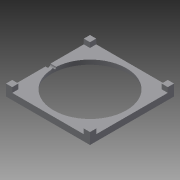
# Autodesk Inventor part: lamp_holder_v1
Saved by Autodesk Inventor 2015 (Build 190159000, 159)
## iProperties
Created: 2021-08-24
Part Number: lamp_holder_v1
Material: Genérico
Document SubType Name: Modeling
Designer: Zuloaga
Density: 1 g/cm^3
Appearance: Valor por defecto
Author: Zuloaga
Autodesk Inventor part; units mm, degrees
ref_plane "YZ Plane" through (0, 0, 0) normal (1, 0, 0) x (0, 1, 0)
ref_plane "XZ Plane" through (0, 0, 0) normal (0, 1, 0) x (-1, 0, 0)
ref_plane "XY Plane" through (0, 0, 0) normal (0, 0, 1) x (1, 0, 0)
sketch "Boceto1" plane through (0, 0, 0) normal (0, 0, 1) x (1, 0, 0)
  circle A0 centre (0, 0) radius 62.5
  line L0 (62.5, 0) -> (67.5, 0)
  line L1 (0, 62.5) -> (0, 67.5)
  line L2 (0, 62.5) -> (5, 62.5) construction
  line L3 (0, 67.5) -> (67.5, 67.5)
  line L4 (67.5, 67.5) -> (67.5, 0)
  line L5 (-62.5, 0) -> (-67.5, 0)
  line L6 (-62.5, 0) -> (-57.5, 0) construction
  line L7 (0, -62.5) -> (0, -67.5)
  line L8 (0, -62.5) -> (5, -62.5) construction
  line L9 (0, -67.5) -> (-67.5, -67.5)
  line L10 (-67.5, -67.5) -> (67.5, -67.5)
  line L11 (67.5, -67.5) -> (67.5, 67.5)
  line L12 (67.5, 67.5) -> (-67.5, 67.5)
  line L13 (-67.5, 67.5) -> (-67.5, -67.5)
  dimension "d0" = 125
  dimension "d1" = 5
  dimension "d2" = 5
  dimension "d3" = 90
  dimension "d4" = 90
  dimension "d5" = 5
  dimension "d6" = 180
  dimension "d7" = 5
  dimension "d8" = 90
  dimension "d9" = 90
  constraints: 28 end point, 6 horizontal, 4 point on circle, 3 equal length, 2 parallel, 2 perpendicular, 2 vertical, 1 centre point, 1 coincident
  measures "d0" diameter of A0
  measures "d1" distance of L0.start L0.end
  measures "d2" distance of L1.start L1.end
  measures "d3" angle of L2 L1
  measures "d4" angle of L1 L3
  measures "d5" distance of L5.start L5.end
  measures "d6" angle of L5 L6
  measures "d7" distance of L7.start L7.end
  measures "d8" angle of L7 L8
  measures "d9" angle of L7 L9
extrude "Extrusión1" add sketch "Boceto1" along normal blind 7 contours L0 L11 L10 L7 A0 | A0 L1 L3 L4 L0 | A0 L5 L13 L12 L1 | L7 L9 L13 L5 A0
sketch "Boceto2" plane through (0, 0, 7) normal (0, 0, 1) x (1, 0, 0)
  line L0 (-67.5, 67.5) -> (67.5, 67.5)
  line L1 (67.5, 67.5) -> (67.5, -67.5)
  line L2 (67.5, -67.5) -> (-67.5, -67.5)
  line L3 (-67.5, -67.5) -> (-67.5, 67.5)
  circle A0 centre (0, 0) radius 58.5
  dimension "d12" = 117
  constraints: 8 end point, 2 parallel, 1 centre point, 1 coincident, 1 horizontal, 1 perpendicular
  measures "d12" diameter of A0
extrude "Extrusión2" add sketch "Boceto2" along normal blind 3
sketch "Boceto3" plane through (0, 0, 10) normal (0, 0, 1) x (1, 0, 0)
  line L0 (-67.5, -67.5) -> (-57.5, -67.5)
  line L1 (-57.5, -67.5) -> (-57.5, -57.5)
  line L2 (-57.5, -57.5) -> (-67.5, -57.5)
  line L3 (-67.5, -57.5) -> (-67.5, -67.5)
  line L4 (67.5, 67.5) -> (57.5, 67.5)
  line L5 (57.5, 67.5) -> (57.5, 57.5)
  line L6 (57.5, 57.5) -> (67.5, 57.5)
  line L7 (67.5, 57.5) -> (67.5, 67.5)
  line L8 (-67.5, 67.5) -> (-57.5, 67.5)
  line L9 (-57.5, 67.5) -> (-57.5, 57.5)
  line L10 (-57.5, 57.5) -> (-67.5, 57.5)
  line L11 (-67.5, 57.5) -> (-67.5, 67.5)
  line L12 (67.5, -67.5) -> (57.5, -67.5)
  line L13 (57.5, -67.5) -> (57.5, -57.5)
  line L14 (57.5, -57.5) -> (67.5, -57.5)
  line L15 (67.5, -57.5) -> (67.5, -67.5)
  point P0 (0, 0)
  dimension "d15" = 10
  dimension "d16" = 10
  dimension "d17" = 10
  dimension "d18" = 10
  dimension "d19" = 10
  dimension "d20" = 10
  dimension "d21" = 10
  dimension "d22" = 10
  constraints: 32 end point, 8 parallel, 4 horizontal, 4 perpendicular
  measures "d15" distance of L2.end L1.end
  measures "d16" distance of L1.end L0.end
  measures "d17" distance of L6.end L5.end
  measures "d18" distance of L5.end L4.end
  measures "d19" distance of L9.end L10.end
  measures "d20" distance of L8.end L9.end
  measures "d21" distance of L13.end L14.end
  measures "d22" distance of L12.end L13.end
extrude "Extrusión3" add sketch "Boceto3" along normal blind 8
sketch "Boceto4" plane through (-67.5, -67.5, 0) normal (-1, 0, 0) x (0, 0, 1)
  line L0 (0, 67.5) -> (10, 67.5)
  line L1 (10, 10) -> (10, 125) projected
  line L2 (10, 67.5) -> (10, 71.5)
  line L3 (10, 67.5) -> (14, 67.5) construction
  line L4 (10, 67.5) -> (10, 63.5)
  line L5 (10, 67.5) -> (14, 67.5) construction
  line L6 (10, 67.5) -> (6, 67.5)
  arc A0 (10, 71.5) -> (10, 63.5) centre (10, 67.5) ccw
  dimension "d25" = 4
  dimension "d26" = 90
  dimension "d27" = 4
  dimension "d28" = 90
  dimension "d29" = 4
  constraints: 12 end point, 3 point on circle, 2 collinear, 2 horizontal, 2 perpendicular, 1 centre point, 1 midpoint, 1 point on line
  measures "d25" distance of L0.end L2.end
  measures "d26" angle of L3 L2
  measures "d27" distance of L0.end L4.end
  measures "d28" angle of L4 L5
  measures "d29" distance of L0.end L6.end
extrude "Extrusión4" cut sketch "Boceto4" against normal blind 10
